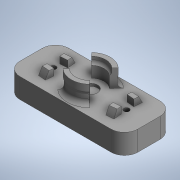
# Autodesk Inventor part: MG996R Arm Test
Saved by Autodesk Inventor 2020.5 (Build 245400000, 400)
## iProperties
Created: 2023-03-16
Part Number: MG996R Arm Test
Material: Generic
Document SubType Name: Modeling
Designer: Wes
Density: 1 g/cm^3
Appearance: Default
Author: Wes
Autodesk Inventor part; units mm, degrees
ref_plane "YZ Plane" through (0, 0, 0) normal (1, 0, 0) x (0, 1, 0)
ref_plane "XZ Plane" through (0, 0, 0) normal (0, 1, 0) x (-1, 0, 0)
ref_plane "XY Plane" through (0, 0, 0) normal (0, 0, 1) x (1, 0, 0)
sketch "Base" plane through (0, 0, 0) normal (0, 0, 1) x (1, 0, 0)
  line L0 (0, 0) -> (-22, 0)
  line L1 (-22, 0) -> (-22, 53)
  line L2 (-22, 53) -> (0, 53)
  line L3 (0, 53) -> (0, 0)
  line L4 (-11, 26.5) -> (-11, 43.6) construction
  line L5 (-11, 26.5) -> (-11, 9.4) construction
  line L6 (-11, 26.5) -> (-11, 10.7) construction
  line L7 (-11, 26.5) -> (-11, 42.3) construction
  line L8 (-11, 10.7) -> (-11, 9.4) construction
  line L9 (-11, 42.3) -> (-11, 43.6) construction
  circle A0 centre (-11, 42.95) radius 1.175
  circle A1 centre (-11, 10.05) radius 1.175
  dimension "d0" = 22
  dimension "d1" = 53
  dimension "d8" = 34.2
  dimension "d14" = 31.6
  dimension "d15" = 2.35
  dimension "d16" = 2.35
  constraints: 20 end point, 3 vertical, 2 centre point, 2 midpoint, 2 parallel, 2 point on line, 1 collinear, 1 horizontal, 1 perpendicular
  measures "d0" distance of L1.end L2.end
  measures "d1" distance of L0.end L1.end
  measures "d8" distance of L4.end L5.end
  measures "d14" distance of L7.end L6.end
  measures "d15" diameter of A0
  measures "d16" diameter of A1
extrude "Extrusion1" add sketch "Base" along normal mid plane 9
sketch "Countersink Arm Screw Holes" plane through (0, 0, -4.5) normal (0, 0, -1) x (-1, 0, 0)
  circle A0 centre (11, 10.05) radius 1.175 projected
  circle A1 centre (11, 10.05) radius 2.7
  circle A2 centre (11, 42.95) radius 1.175 projected
  circle A3 centre (11, 42.95) radius 2.7
  point P0 (0, 0)
  dimension "d19" = 5.4
  dimension "d20" = 5.4
  constraints: 2 centre point, 2 coincident
  measures "d19" diameter of A1
  measures "d20" diameter of A3
extrude "Extrusion2" cut sketch "Countersink Arm Screw Holes" against normal blind 1.8 contours A0 | A1 | A2 | A3
sketch "Axle Screw Countersink" plane through (0, 0, 4.5) normal (0, 0, 1) x (1, 0, 0)
  circle A0 centre (-11.089431, 26.715447) radius 3.1
  point P0 (0, 0)
  dimension "d23" = 6.2
  constraints: 1 centre point
  measures "d23" diameter of A0
extrude "Extrusion3" cut sketch "Axle Screw Countersink" against normal blind 1.2
sketch "Arm Center Fitting" plane through (0, 0, 4.5) normal (0, 0, 1) x (1, 0, 0)
  circle A0 centre (-11.089431, 26.715447) radius 5.975 construction
  line L0 (-6.696468, 22.665447) -> (-6.696468, 30.765447) construction
  line L1 (-6.696468, 22.665447) -> (-15.482394, 22.665447) construction
  line L2 (-15.482394, 22.665447) -> (-15.482394, 30.765447) construction
  arc A1 (-15.482394, 30.765447) -> (-15.482394, 22.665447) centre (-11.089431, 26.715447) ccw
  line L3 (-15.482394, 22.665447) -> (-17.320454, 20.970886)
  line L4 (-15.482394, 30.765447) -> (-17.320454, 32.460008)
  arc A2 (-17.320454, 32.460008) -> (-17.320454, 20.970886) centre (-11.089431, 26.715447) ccw
  line L5 (-11.089431, 16.056342) -> (-11.089431, 38.404771) construction
  arc A3 (-6.696468, 22.665447) -> (-6.696468, 30.765447) centre (-11.089431, 26.715447) ccw
  line L6 (-6.696468, 22.665447) -> (-4.858408, 20.970886)
  line L7 (-6.696468, 30.765447) -> (-4.858408, 32.460008)
  arc A4 (-4.858408, 20.970886) -> (-4.858408, 32.460008) centre (-11.089431, 26.715447) ccw
  point P0 (0, 0)
  dimension "d27" = 11.95
  dimension "d31" = 8.1
  dimension "d32" = 8.1
  dimension "d33" = 2.5
  dimension "d34" = 2.5
  constraints: 16 end point, 12 point on circle, 5 centre point, 2 line through centre, 2 symmetric about line, 2 vertical, 1 coincident, 1 concentric, 1 perpendicular, 2 other
  measures "d27" diameter of A0
  measures "d31" distance of L0.start L0.end
  measures "d32" distance of L1.end L2.end
  measures "d33" distance of L1.end L3.end
  measures "d34" distance of L2.end L4.end
extrude "Extrusion4" add sketch "Arm Center Fitting" along normal blind 5
sketch "Rotation Support" plane through (0, 0, 9.5) normal (0, 0, 1) x (1, 0, 0)
  line L0 (-17.064431, 26.715447) -> (-17.864431, 26.715447) construction
  circle A0 centre (-11.089431, 26.715447) radius 6.775 construction
  arc A1 (-16.070573, 31.307707) -> (-16.070573, 22.123188) centre (-11.089431, 26.715447) ccw
  line L1 (-17.864431, 26.715447) -> (-19.864431, 26.715447) construction
  circle A2 centre (-11.089431, 26.715447) radius 8.775 construction
  arc A3 (-17.541021, 32.663355) -> (-17.541021, 20.767539) centre (-11.089431, 26.715447) ccw
  line L2 (-17.541021, 20.767539) -> (-16.070573, 22.123188)
  line L3 (-15.482394, 22.665447) -> (-17.320454, 20.970886)
  line L4 (-16.070573, 31.307707) -> (-17.541021, 32.663355)
  line L5 (-17.320454, 32.460008) -> (-15.482394, 30.765447)
  line L6 (-11.089431, 15.244922) -> (-11.089431, 38.763368) construction
  arc A4 (-6.108289, 22.123188) -> (-6.108289, 31.307707) centre (-11.089431, 26.715447) ccw
  arc A5 (-4.637841, 20.767539) -> (-4.637841, 32.663355) centre (-11.089431, 26.715447) ccw
  line L7 (-4.637841, 20.767539) -> (-6.108289, 22.123188)
  line L8 (-6.108289, 31.307707) -> (-4.637841, 32.663355)
  point P0 (0, 0)
  dimension "d38" = 0.8
  dimension "d39" = 2
  constraints: 16 point on circle, 14 end point, 6 centre point, 4 symmetric about line, 2 coincident, 2 collinear, 2 horizontal, 1 concentric, 1 vertical, 2 other
  measures "d38" distance of L0.start L0.end
  measures "d39" distance of L0.end L1.end
extrude "Extrusion5" add sketch "Rotation Support" along normal blind 3
sketch "Arm Support" plane through (0, 0, 4.5) normal (0, 0, 1) x (1, 0, 0)
  circle A0 centre (-11, 10.05) radius 1.175 construction
  line L0 (-11, 8.875) -> (-11, 13.375) construction
  line L1 (-11, 10.05) -> (-13.85, 10.05) construction
  line L2 (-11, 10.05) -> (-8.15, 10.05) construction
  line L3 (-11, 13.375) -> (-7.875, 13.375) construction
  line L4 (-11, 13.375) -> (-14.125, 13.375) construction
  line L5 (-13.85, 10.05) -> (-14.125, 13.375)
  line L6 (-14.125, 13.375) -> (-16.118194, 13.210149)
  line L7 (-16.118194, 13.210149) -> (-15.843194, 9.885149)
  line L8 (-15.843194, 9.885149) -> (-13.85, 10.05)
  line L9 (-8.15, 10.05) -> (-7.875, 13.375)
  line L10 (-7.875, 13.375) -> (-5.881806, 13.210149)
  line L11 (-5.881806, 13.210149) -> (-6.156806, 9.885149)
  line L12 (-6.156806, 9.885149) -> (-8.15, 10.05)
  line L13 (-17.064431, 26.715447) -> (-5.114431, 26.715447) construction
  line L14 (-13.85, 43.380894) -> (-14.125, 40.055894)
  line L15 (-14.125, 40.055894) -> (-16.118194, 40.220745)
  line L16 (-16.118194, 40.220745) -> (-15.843194, 43.545745)
  line L17 (-15.843194, 43.545745) -> (-13.85, 43.380894)
  line L18 (-8.15, 43.380894) -> (-7.875, 40.055894)
  line L19 (-6.156806, 43.545745) -> (-8.15, 43.380894)
  line L20 (-7.875, 40.055894) -> (-5.881806, 40.220745)
  line L21 (-5.881806, 40.220745) -> (-6.156806, 43.545745)
  point P0 (0, 0)
  dimension "d45" = 4.5
  dimension "d48" = 5.7
  dimension "d51" = 6.25
  dimension "d52" = 2
  constraints: 44 end point, 10 symmetric about line, 5 horizontal, 2 perpendicular, 1 vertical, 1 vertical alignment, 1 other
  measures "d45" distance of L0.start L0.end
  measures "d48" distance of L1.end L2.end
  measures "d51" distance of L4.end L3.end
  measures "d52" distance of L4.end L6.end
extrude "Extrusion6" add sketch "Arm Support" along normal blind 3
draft "FaceDraft1" angle 28 pull direction (0, 0, 1) faces at (-6.065139, 10.993483, 5.5) (-5.973472, 41.329078, 5.5) fixed edges at (-6.019306, 11.547649, 7.5) (-6.019306, 41.883245, 7.5)
draft "FaceDraft2" angle 28 pull direction (0, 0, 1) faces at (-16.026528, 12.101816, 5.5) (-15.934861, 42.437412, 5.5) fixed edges at (-15.980694, 11.547649, 7.5) (-15.980694, 41.883245, 7.5)
fillet "Fillet1" radius 2 6 edges at (-17.8644, 26.7154, 9.5) (-4.3144, 26.7154, 9.5) (-19.5644, 26.7154, 4.5) (-2.6144, 26.7154, 4.5) (-19.5644, 26.7154, 9.5) (-2.6144, 26.7154, 9.5)
fillet "Fillet2" radius 6 4 edges at (0, 0, 0) (0, 53, 0) (-22, 53, 0) (-22, 0, 0)
body "Solid1"
